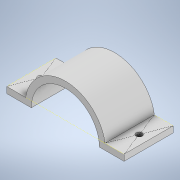
# Autodesk Inventor part: ShootingMech_MotorMount
Saved by Autodesk Inventor 2020 (Build 240168000, 168)
## iProperties
Created: 2022-01-28
Part Number: ShootingMech_MotorMount
Material: Generic
Document SubType Name: Modeling
Designer: danie
Density: 1 g/cm^3
Appearance: Default
Author: danie
Autodesk Inventor part; units mm, degrees
ref_plane "YZ Plane" through (0, 0, 0) normal (1, 0, 0) x (0, 1, 0)
ref_plane "XZ Plane" through (0, 0, 0) normal (0, 1, 0) x (-1, 0, 0)
ref_plane "XY Plane" through (0, 0, 0) normal (0, 0, 1) x (1, 0, 0)
sketch "Sketch1" plane through (0, 0, 0) normal (0, 0, 1) x (1, 0, 0)
  arc A0 (17.526, 0) -> (-17.526, 0) centre (0, 0) ccw
  arc A1 (20.701, 0) -> (-20.701, 0) centre (0, 0) ccw
  line L0 (17.526, 0) -> (30.226, 0)
  line L1 (30.226, 0) -> (30.226, 3.175)
  line L2 (30.226, 3.175) -> (17.526, 3.175)
  line L3 (17.526, 3.175) -> (17.526, 0)
  line L4 (-17.526, 0) -> (-30.226, 0)
  line L5 (-30.226, 0) -> (-30.226, 3.175)
  line L6 (-30.226, 3.175) -> (-17.526, 3.175)
  line L7 (-17.526, 3.175) -> (-17.526, 0)
  point P0 (20.4561, 3.175)
  point P1 (-20.4561, 3.175)
  dimension "d0" = 17.526
  dimension "d1" = 3.175
  dimension "d2" = 12.7
  dimension "d3" = 3.175
  dimension "d4" = 12.7
  dimension "d5" = 3.175
  constraints: 16 end point, 4 parallel, 4 point on circle, 2 centre point, 2 horizontal, 2 perpendicular, 1 coincident
  measures "d0" radius of A0
  measures "d1" radial gap between concentric circles of A0 A1
  measures "d2" distance of L2.end L1.end
  measures "d3" distance of L1.end L0.end
  measures "d4" distance of L5.end L6.end
  measures "d5" distance of L4.end L5.end
extrude "Extrusion1" add sketch "Sketch1" along normal blind 25.4
sketch "Sketch2" plane through (-30.226, 3.175, 0) normal (0, 1, 0) x (1, 0, 0)
  line L0 (0, 0) -> (0, -25.4) construction
  line L1 (9.7699, 0) -> (50.6821, 0) construction
  line L2 (0, -25.4) -> (9.7699, 0) construction
  line L3 (9.7699, -25.4) -> (50.6821, -25.4) construction
  line L4 (0, 0) -> (9.7699, -25.4) construction
  line L5 (47.752, 0) -> (60.452, 0) construction
  line L6 (50.6821, -25.4) -> (60.452, 0) construction
  line L7 (47.752, -25.4) -> (60.452, -25.4) construction
  line L8 (60.452, -25.4) -> (50.6821, 0) construction
  point P0 (30.226, 0)
  constraints: 8 end point
sketch "Sketch3" plane through (-30.226, 3.175, 0) normal (0, 1, 0) x (1, 0, 0)
  point P0 (30.226, 0)
  point P1 (4.885, -12.7)
hole "Hole1" at (-25.341, 3.175, 12.7) direction (0, -1, 0) diameter 3.175 end through all
sketch "Sketch4" plane through (20.4561, 3.175, 0) normal (0, 1, 0) x (1, 0, 0)
  point P0 (-20.4561, 0)
  point P1 (4.885, -12.7)
hole "Hole2" at (25.341, 3.175, 12.7) direction (0, -1, 0) diameter 3.175 end through all
body "Solid1"
